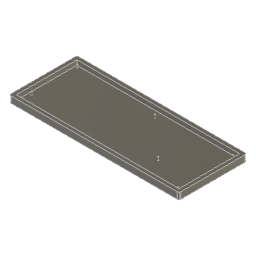
StreamForge-Full (Autodesk Fusion 360 archive; units mm, degrees)
design "Streamforge-Case"
part number: 2026-03-29-16-38-54-488
Autodesk Fusion 360 part; units mm, degrees
sketch "Sketch1" plane through (0, 0, 0) normal (0, 0, 1) x (1, 0, 0)
  line L0 (-100, 50) -> (346.68, 50)
  line L1 (346.68, 50) -> (346.68, -116.26)
  line L2 (346.68, -116.26) -> (-100, -116.26)
  line L3 (-100, -116.26) -> (-100, 50)
  line L4 (-110, 60) -> (356.68, 60)
  line L5 (356.68, 60) -> (356.68, -126.26)
  line L6 (356.68, -126.26) -> (-110, -126.26)
  line L7 (-110, -126.26) -> (-110, 60)
  dimension "d1" = 446.68
  dimension "d2" = 166.26
  dimension "d3" = 466.68
  dimension "d4" = 186.26
  dimension "d5" = 10
  dimension "d6" = 10
  constraint horizontal L0
  constraint vertical L1
  constraint horizontal L2
  constraint vertical L3
  constraint horizontal L4
  constraint vertical L5
  constraint horizontal L6
  constraint vertical L7
  measures "d1" distance of L0.start L0.end
  measures "d2" distance of L0.start L2.end
  measures "d3" distance of L4.start L4.end
  measures "d4" distance of L4.start L6.end
  measures "d5" distance of L0 L4
  measures "d6" distance of L3 L7
extrude "Extrude1" add sketch "Sketch1" along normal blind 5 contours L0 L1 L2 L3
extrude "Extrude2" add sketch "Sketch1" along normal blind 18
sketch "Sketch2" plane through (0, 0, 5) normal (0, 0, 1) x (-1, 0, 0)
  line L0 (100, 116.26) -> (-346.68, 116.26)
  line L1 (-346.68, 116.26) -> (-346.68, -50)
  line L2 (-346.68, -50) -> (100, -50)
  line L3 (100, -50) -> (100, 116.26)
  circle A0 centre (94, -45.04) radius 1.7
  circle A1 centre (-132.22, -32.1) radius 1.7
  circle A2 centre (92.07, 82.66) radius 1.7
  circle A3 centre (-95.96, 112.43) radius 1.7
  circle A4 centre (-237.26, 64.33) radius 1.7
  circle A5 centre (-335.42, -43.13) radius 1.7
  circle A6 centre (-336.97, 108.98) radius 1.7
  line L4 (100, -50) -> (-346.68, -50)
  line L5 (100, 116.26) -> (100, -50)
  line L6 (-346.68, 116.26) -> (100, 116.26)
  line L7 (-346.68, -50) -> (-346.68, 116.26)
  dimension "d11" = 3.4
  dimension "d12" = 3.4
  dimension "d13" = 3.4
  dimension "d14" = 3.4
  dimension "d15" = 3.4
  dimension "d16" = 3.4
  dimension "d17" = 3.4
  dimension "d18" = 4.96
  dimension "d19" = 6
  dimension "d20" = 7.93
  dimension "d21" = 33.6
  dimension "d22" = 195.96
  dimension "d23" = 3.83
  dimension "d24" = 109.42
  dimension "d25" = 51.93
  dimension "d26" = 7.28
  dimension "d27" = 9.71
  dimension "d28" = 11.26
  dimension "d29" = 6.87
  dimension "d30" = 214.46
  dimension "d31" = 17.9
  measures "d11" diameter of A0
  measures "d12" diameter of A1
  measures "d13" diameter of A2
  measures "d14" diameter of A3
  measures "d15" diameter of A4
  measures "d16" diameter of A5
  measures "d17" diameter of A6
  measures "d18" distance of A0.centre L4
  measures "d19" distance of A0.centre L5
  measures "d20" distance of A2.centre L5
  measures "d21" distance of A2.centre L6
  measures "d22" distance of A3.centre L5
  measures "d23" distance of A3.centre L6
  measures "d24" distance of A4.centre L7
  measures "d25" distance of A4.centre L6
  measures "d26" distance of A6.centre L6
  measures "d27" distance of A6.centre L7
  measures "d28" distance of A5.centre L7
  measures "d29" distance of A5.centre L4
  measures "d30" distance of A1.centre L7
  measures "d31" distance of A1.centre L4
extrude "Extrude3" add sketch "Sketch2" along normal blind 8 contours A0 | A1 | A2 | A3 | A4 | A5 | A6
fillet "Fillet1" radius 5 4 edges at (356.68, -126.26, 9) (356.68, 60, 9) (-110, 60, 9) (-110, -126.26, 9)
